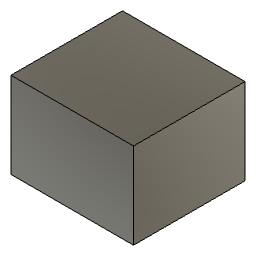
just_a_cube v1 Test_upload (Autodesk Fusion 360 design; units mm, degrees)
Autodesk Fusion 360 part; units mm, degrees
sketch "Sketch1" plane through (0, 0, 0) normal (0, 0, 1) x (1, 0, 0)
  line L0 (-31.4264, 31.6402) -> (47.0327, 31.6402)
  line L1 (47.0327, 31.6402) -> (47.0327, -39.764)
  line L2 (47.0327, -39.764) -> (-31.4264, -39.764)
  line L3 (-31.4264, -39.764) -> (-31.4264, 31.6402)
  constraint horizontal L0
  constraint vertical L1
  constraint horizontal L2
  constraint vertical L3
extrude "Extrude1" add sketch "Sketch1" along normal blind 55
